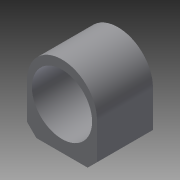
# Autodesk Inventor part: x bushing holder full
Saved by Autodesk Inventor 2014 SP1 (Build 180222100, 222)
## iProperties
Created: 2014-10-23
Part Number: x bushing holder full
Material: Generic
Document SubType Name: Modeling
Designer: Mon
Density: 1 g/cm^3
Appearance: Default
Author: Mon
Autodesk Inventor part; units mm, degrees
ref_plane "YZ Plane" through (0, 0, 0) normal (1, 0, 0) x (0, 1, 0)
ref_plane "XZ Plane" through (0, 0, 0) normal (0, 1, 0) x (-1, 0, 0)
ref_plane "XY Plane" through (0, 0, 0) normal (0, 0, 1) x (1, 0, 0)
sketch "Sketch1" plane through (0, 0, 0) normal (0, 1, 0) x (-1, 0, 0)
  circle A0 centre (0, 0) radius 6.45
  arc A1 (7.5, 0.8257) -> (-7.5, 0.8257) centre (0, 0.8257) ccw
  line L0 (-7.5, -5.5743) -> (-7.5, 0.8257)
  line L1 (7.5, -5.5743) -> (7.5, 0.8257)
  line L2 (7.5, -5.5743) -> (7.5, -9)
  line L3 (-7.5, -5.5743) -> (-7.5, -9)
  line L4 (7.5, -9) -> (-7.5, -9)
  dimension "d0" = 12.9
  dimension "d2" = 7.5
  dimension "d7" = 9
  constraints: 10 end point, 2 centre point, 2 point on circle, 2 tangent, 1 coincident, 1 collinear, 1 parallel, 1 perpendicular, 1 vertical
  measures "d0" diameter of A0
  measures "d2" radius of A1
  measures "d7" distance from line of L4 point (0, 0)
extrude "Extrusion1" add sketch "Sketch1" along normal blind 12
chamfer "Chamfer1" distance 2 angle 45 1 edges at (7.5, 6, -9)
chamfer "Chamfer2" distance 2 angle 45 1 edges at (-7.5, 6, -9)
body "Solid1"
